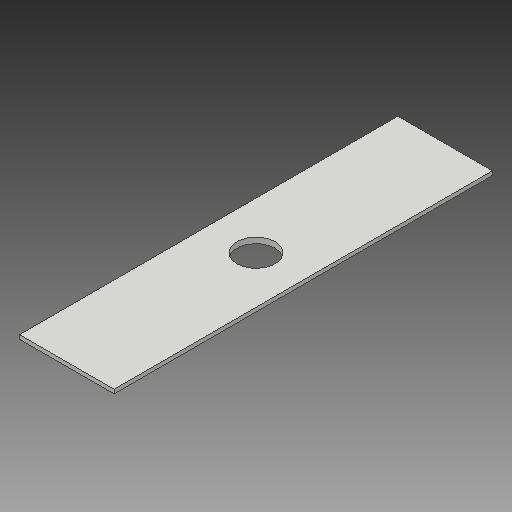
# Autodesk Inventor part: Tapa
Saved by Autodesk Inventor 2017 (Build 210142000, 142)
## iProperties
Created: 2017-01-19
Part Number: Tapa
Material: Generic
Document SubType Name: Modeling
Designer: A. Matías Quezada
Density: 1 g/cm^3
Appearance: Default
Author: A. Matías Quezada
Autodesk Inventor part; units mm, degrees
ref_plane "YZ Plane" through (0, 0, 0) normal (1, 0, 0) x (0, 1, 0)
ref_plane "XZ Plane" through (0, 0, 0) normal (0, 1, 0) x (-1, 0, 0)
ref_plane "XY Plane" through (0, 0, 0) normal (0, 0, 1) x (1, 0, 0)
sketch "Sketch1" plane through (0, 0, 0) normal (0, 0, 1) x (1, 0, 0)
  line L0 (0, 0) -> (-200, 0)
  line L1 (-200, 0) -> (-200, 50)
  line L2 (-200, 50) -> (0, 50)
  line L3 (0, 50) -> (0, 0)
  dimension "d0" = 200
  dimension "d1" = 50
  constraints: 8 end point, 2 parallel, 1 horizontal, 1 perpendicular
  measures "d0" distance of L1.end L2.end
  measures "d1" distance of L0.end L1.end
extrude "Cuerpo" add sketch "Sketch1" along normal blind 2.1
sketch "Sketch2" plane through (0, 0, 0) normal (0, 0, -1) x (-1, 0, 0)
  line L0 (0, 0) -> (200, 0) projected
  line L1 (200, 0) -> (200, 50) projected
  line L2 (200, 50) -> (0, 50) projected
  line L3 (0, 50) -> (0, 0) projected
  line L4 (0, 0) -> (200, 0) projected
  line L5 (200, 0) -> (200, 50) projected
  line L6 (200, 50) -> (0, 50) projected
  line L7 (0, 50) -> (0, 0) projected
  line L8 (196.8, 3.2) -> (3.2, 3.2)
  line L9 (3.2, 3.2) -> (3.2, 46.8)
  line L10 (3.2, 46.8) -> (196.8, 46.8)
  line L11 (196.8, 46.8) -> (196.8, 3.2)
  dimension "d4" = 3.2
  constraints: 8 end point, 3 other
  measures "d4" distance between parallel lines of L0 L8
extrude "Ranura" add sketch "Sketch2" along normal blind 0.9 contours L8 L9 L10 L11
sketch "Sketch4" plane through (0, 0, 2.1) normal (0, 0, 1) x (1, 0, 0)
  line L0 (-200, 50) -> (0, 50) projected
  line L1 (-100, 50) -> (-100, 0)
  line L2 (-200, 0) -> (0, 0) projected
  point P0 (-100, 25)
  constraints: 3 midpoint, 2 end point
hole "Rueda Externa" at (-100, 25, 2.1) direction (0, 0, -1) diameter 20.2 end through all
equation "\"d0\" = base_largo"
equation "\"d1\" = base_ancho"
equation "\"d2\" = tapa_grosor"
equation "\"d4\" = base_muros_grosor + general_margen"
equation "\"d5\" = tapa_ranura"
equation "\"d8\" = tapa_eje_diametro"
equation "\"base_largo\" = 200"
equation "\"base_ancho\" = 50"
equation "\"tapa_grosor\" = 2.1"
equation "\"base_muros_grosor\" = 3"
equation "\"general_margen\" = 0.2"
equation "\"tapa_ranura\" = 0.9"
equation "\"tapa_eje_diametro\" = 20.2"
body "Solid1"
